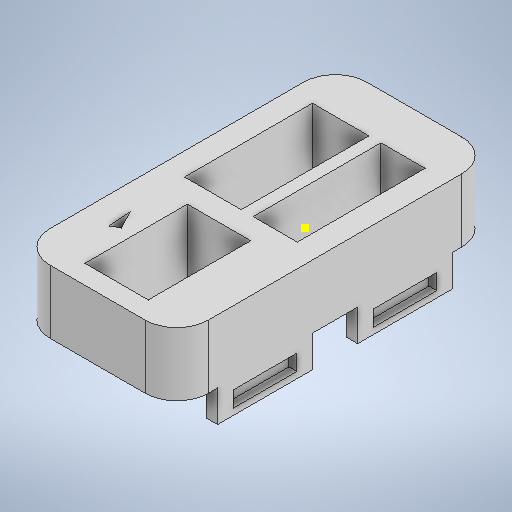
# Autodesk Inventor part: Testing
Saved by Autodesk Inventor 2025.1 (Build 291241000, 241)
## iProperties
Created: 2025-08-26
Part Number: Testing
Material: Generic
Document SubType Name: Modeling
Designer: eugen
Density: 1 g/cm^3
Appearance: Default
Author: eugen
Autodesk Inventor part; units mm, degrees
ref_plane "YZ Plane" through (0, 0, 0) normal (1, 0, 0) x (0, 1, 0)
ref_plane "XZ Plane" through (0, 0, 0) normal (0, 1, 0) x (-1, 0, 0)
ref_plane "XY Plane" through (0, 0, 0) normal (0, 0, 1) x (1, 0, 0)
sketch "Sketch1" plane through (0, 0, 0) normal (0, 1, 0) x (-1, 0, 0)
  line L0 (29.9672, 50.4505) -> (-0.0328, 50.4505)
  line L1 (-10.0328, 40.4505) -> (-10.0328, -39.5495)
  line L2 (-0.0328, -49.5495) -> (29.9672, -49.5495)
  line L3 (39.9672, -39.5495) -> (39.9672, 40.4505)
  line L4 (24.9672, 44.4505) -> (4.9672, 44.4505)
  line L5 (4.9672, 44.4505) -> (4.9672, 12.105)
  line L6 (4.9672, 12.105) -> (24.9672, 12.105)
  line L7 (24.9672, 12.105) -> (24.9672, 44.4505)
  line L8 (32.8329, 5.1351) -> (14.9672, 5.1351)
  line L9 (14.9672, 5.1351) -> (14.9672, -35.2063)
  line L10 (14.9672, -35.2063) -> (32.8329, -35.2063)
  line L11 (32.8329, -35.2063) -> (32.8329, 5.1351)
  line L12 (11.1837, 5.1351) -> (-2.7562, 5.1351)
  line L13 (-2.7562, 5.1351) -> (-2.7562, -35.2063)
  line L14 (-2.7562, -35.2063) -> (11.1837, -35.2063)
  line L15 (11.1837, -35.2063) -> (11.1837, 5.1351)
  arc A0 (-0.0328, 50.4505) -> (-10.0328, 40.4505) centre (-0.0328, 40.4505) ccw
  arc A1 (39.9672, 40.4505) -> (29.9672, 50.4505) centre (29.9672, 40.4505) ccw
  arc A2 (29.9672, -49.5495) -> (39.9672, -39.5495) centre (29.9672, -39.5495) ccw
  arc A3 (-10.0328, -39.5495) -> (-0.0328, -49.5495) centre (-0.0328, -39.5495) ccw
  point P0 (0, 0)
  point P1 (39.9672, 50.4505)
  point P2 (-10.0328, -49.5495)
  point P3 (39.9672, -49.5495)
  dimension "d1" = 100
  dimension "d2" = 50
  dimension "d3" = 15
  dimension "d4" = 15
  dimension "d6" = 6
  dimension "d7" = 10
  dimension "d8" = 10
  dimension "d9" = 10
  dimension "d10" = 10
  constraints: 32 end point, 8 parallel, 8 point on circle, 8 point on line, 8 tangent, 4 centre point, 4 horizontal, 4 perpendicular
  measures "d1" distance of point (39.967, -49.55) point (39.967, 50.45)
  measures "d2" distance of point (-10.033, -49.55) point (39.967, -49.55)
  measures "d3" distance between parallel lines of L3 L7
  measures "d4" distance between parallel lines of L1 L5
  measures "d6" distance between parallel lines of L0 L4
  measures "d7" radius of A0
  measures "d8" radius of A1
  measures "d9" radius of A2
  measures "d10" radius of A3
extrude "Extrusion1" add sketch "Sketch1" along normal blind 20
sketch "Sketch2" plane through (0, 0, 0) normal (0, -1, 0) x (1, 0, 0)
  line L0 (10.0328, 40.4505) -> (10.0328, -39.5495) projected
  line L1 (10.0328, 37.5913) -> (6.5328, 37.5913)
  line L2 (6.5328, 37.5913) -> (6.5328, 7.5913)
  line L3 (6.5328, 7.5913) -> (10.0328, 7.5913)
  line L4 (10.0328, 7.5913) -> (10.0328, 37.5913)
  line L5 (10.0328, -6.6206) -> (6.5328, -6.6206)
  line L6 (6.5328, -6.6206) -> (6.5328, -36.6206)
  line L7 (6.5328, -36.6206) -> (10.0328, -36.6206)
  line L8 (10.0328, -36.6206) -> (10.0328, -6.6206)
  arc A0 (10.0328, 40.4505) -> (0.0328, 50.4505) centre (0.0328, 40.4505) ccw projected
  arc A1 (0.0328, -49.5495) -> (10.0328, -39.5495) centre (0.0328, -39.5495) ccw projected
  line L9 (-39.9672, -39.5495) -> (-39.9672, 40.4505) projected
  line L10 (-39.9672, 37.5913) -> (-36.4672, 37.5913)
  line L11 (-36.4672, 37.5913) -> (-36.4672, 7.5913)
  line L12 (-36.4672, 7.5913) -> (-39.9672, 7.5913)
  line L13 (-39.9672, 7.5913) -> (-39.9672, 37.5913)
  line L14 (-39.9672, -6.6206) -> (-36.4672, -6.6206)
  line L15 (-36.4672, -6.6206) -> (-36.4672, -36.6206)
  line L16 (-36.4672, -36.6206) -> (-39.9672, -36.6206)
  line L17 (-39.9672, -36.6206) -> (-39.9672, -6.6206)
  point P0 (0, 0)
  point P1 (7.1038, 47.5215)
  point P2 (8.2828, 37.5913)
  point P3 (7.1038, -46.6206)
  point P4 (8.2828, 7.5913)
  point P5 (-34.5818, 22.0482)
  point P6 (-38.0818, -7.9518)
  point P7 (-37.5107, 76.1904)
  point P8 (-36.4672, -21.6206)
  point P9 (-39.9672, -21.6206)
  dimension "d13" = 3.5
  dimension "d14" = 3.5
  dimension "d15" = 10
  dimension "d16" = 10
  dimension "d17" = 30
  dimension "d18" = 30
  dimension "d22" = 3.5
  dimension "d23" = 3.5
  constraints: 32 end point, 8 parallel, 5 point on line, 4 horizontal, 4 midpoint, 4 perpendicular, 2 point on circle
  measures "d13" distance between parallel lines of L0 L2
  measures "d14" distance between parallel lines of L8 L6
  measures "d15" distance of point (7.104, 47.522) point (8.283, 37.591)
  measures "d16" distance from line of L7 point (7.104, -46.621)
  measures "d17" distance of point (8.283, 37.591) point (8.283, 7.591)
  measures "d18" distance between parallel lines of L7 L5
  measures "d22" distance between parallel lines of L9 L11
  measures "d23" distance of point (-36.467, -21.621) point (-39.967, -21.621)
extrude "Extrusion2" add sketch "Sketch2" along normal blind 10
fillet "Fillet1" radius 2 4 edges at (6.5328, 0, 22.5913) (6.5328, 0, -21.6206) (-36.4672, 0, 22.5913) (-36.4672, 0, -21.6206)
sketch "Sketch3" plane through (10.0328, 0, -39.5495) normal (1, 0, 0) x (0, 0, -1)
  line L0 (-72.1408, -3) -> (-52.1157, -3)
  line L1 (-52.1157, -3) -> (-52.1157, -8)
  line L2 (-52.1157, -8) -> (-72.1408, -8)
  line L3 (-72.1408, -8) -> (-72.1408, -3)
  line L4 (-77.1408, 0) -> (-77.1408, -10) projected
  line L5 (-47.1408, 0) -> (-47.1408, -10) projected
  line L6 (-77.1408, 0) -> (-47.1408, 0) projected
  line L7 (-27.9289, -3) -> (-7.9289, -3)
  line L8 (-7.9289, -3) -> (-7.9289, -8)
  line L9 (-7.9289, -8) -> (-27.9289, -8)
  line L10 (-27.9289, -8) -> (-27.9289, -3)
  line L11 (-32.9289, 0) -> (-32.9289, -10) projected
  line L12 (-2.9289, 0) -> (-2.9289, -10) projected
  point P0 (-39.5495, 0)
  point P1 (-77.1408, -5)
  point P2 (-52.1157, -5.5)
  point P3 (-47.1408, -5)
  point P4 (-32.9289, -5)
  point P5 (-27.9289, -5.5)
  point P6 (-2.9289, -5)
  point P7 (-7.9289, -5.5)
  dimension "d27" = 5
  dimension "d28" = 5
  dimension "d29" = 5
  dimension "d30" = 3
  dimension "d31" = 5
  dimension "d33" = 5
  constraints: 16 end point, 7 midpoint, 4 parallel, 2 horizontal, 2 perpendicular
  measures "d27" distance between parallel lines of L2 L0
  measures "d28" distance from line of point (-77.141, -5) L3
  measures "d29" distance of point (-52.116, -5.5) point (-47.141, -5)
  measures "d30" distance between parallel lines of L6 L0
  measures "d31" horizontal distance of point (-32.929, -5) point (-27.929, -5.5)
  measures "d33" distance from line of point (-7.929, -5.5) L12
extrude "Extrusion3" cut sketch "Sketch3" against normal blind 2.5
sketch "Sketch4" plane through (0, 20, 0) normal (0, 1, 0) x (1, 0, 0)
  point P0 (0, 0)
sketch "Sketch5" plane through (0, 20, 0) normal (0, 1, 0) x (1, 0, 0)
  line L0 (-31.3896, -30.3859) -> (-31.9666, -23.1707)
  line L1 (-31.9666, -23.1707) -> (-28.8346, -29.0171)
  line L2 (-28.8346, -29.0171) -> (-31.3896, -30.3859)
  point P0 (0, 0)
  constraints: 6 end point, 1 perpendicular
extrude "Extrusion4" cut sketch "Sketch5" against normal blind 5
sketch "Sketch6" plane through (-39.9672, 0, 40.4505) normal (-1, 0, 0) x (0, 0, 1)
  line L0 (-47.0711, -2) -> (-77.0711, -2) projected
  line L1 (-72.0711, -2) -> (-52.0711, -2)
  line L2 (-52.0711, -2) -> (-52.0711, -8)
  line L3 (-52.0711, -8) -> (-72.0711, -8)
  line L4 (-72.0711, -8) -> (-72.0711, -2)
  line L5 (-47.0711, 0) -> (-47.0711, -10) projected
  line L6 (-77.0711, 0) -> (-77.0711, -10) projected
  line L7 (-47.0711, -10) -> (-77.0711, -10) projected
  line L8 (-2.8592, -2) -> (-32.8592, -2) projected
  line L9 (-27.8843, -8) -> (-7.8592, -8) projected
  line L10 (-27.8592, -2) -> (-7.8592, -2)
  line L11 (-7.8592, -2) -> (-7.8592, -8)
  line L12 (-7.8592, -8) -> (-27.8592, -8)
  line L13 (-27.8592, -8) -> (-27.8592, -2)
  line L14 (-32.8592, 0) -> (-32.8592, -10) projected
  point P0 (-40.4505, 0)
  point P1 (-47.0711, -5)
  point P2 (-77.0711, -5)
  point P3 (-32.8592, -5)
  point P4 (-27.8592, -5)
  point P5 (-7.8592, -2)
  dimension "d38" = 5
  dimension "d39" = 5
  dimension "d40" = 2
  dimension "d41" = 5
  constraints: 16 end point, 4 midpoint, 4 parallel, 2 horizontal, 2 perpendicular, 2 point on line
  measures "d38" distance from line of L2 point (-47.071, -5)
  measures "d39" distance from line of L4 point (-77.071, -5)
  measures "d40" distance between parallel lines of L3 L7
  measures "d41" distance of point (-32.859, -5) point (-27.859, -5)
extrude "Extrusion5" cut sketch "Sketch6" against normal blind 5 contours L2 L3 L4 L0 | L11 L9 L13 L8
body "Solid1"
